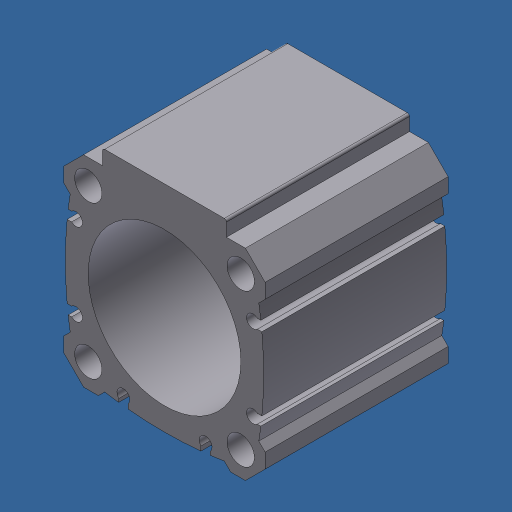
# Autodesk Inventor part: EXTRUSION, CYLINDER, ALUMINIUM, PHD, 50MM
Saved by Autodesk Inventor 2024.3 (Build 283343000, 343)
## iProperties
Manager: _
Category: _
RuleStatus: InUse
Shininess: 64.0
Angle Display Precision: 2
Document Length Units: 11269
Document Angle Units: 11279
Document Time Units: 11290
Document Mass Units: 11283
Document Length Units Precision: 3
Document Angle Units Precision: 2
Part Number: EXTRUSION, CYLINDER, ALUMINIUM, PHD, 50MM
Material: Aluminum, 6061-T6
Document SubType Name: Modeling
Created: 2019-07-31
Designer: -
Manufacturer: Standard
Standards Organization: Custom
Checked By: 00
Engr Approved By: _
User Status: Work In Process
Description: EXTRUSION, CYLINDER, ALUMINIUM, PHD, 50MM
Density: 2.71 g/cm^3
Mass: 328.022 g
Surface Area: 394.618 cm^2
Volume: 121.041 cm^3
Mfg Approved By: -
Appearance: Aluminum (Flat)
BeforeDocSave0: Mass
BeforeDocSave1: PartFinishTrigger
Density: 0.0
Volumn: 0.0
Area: 0.0
PropertySet Name: Model Information
Control State: 0
Master: False
Checked Out: False
CN_MASS: 0.33
CN_SERVICEABLE: _
CL_runCount: 0
FIRST_DESCRIPTION: _
SECOND_DESCRIPTION: _
THIRD_DESCRIPTION: _
Revision Number: A
Subject: _
Author: -
Keywords: -
Autodesk Inventor part; units mm, degrees
ref_plane "YZ Plane" through (0, 0, 0) normal (1, 0, 0) x (0, 1, 0)
ref_plane "XZ Plane" through (0, 0, 0) normal (0, 1, 0) x (-1, 0, 0)
ref_plane "XY Plane" through (0, 0, 0) normal (0, 0, 1) x (1, 0, 0)
sketch "Sketch1" plane through (0, 0, 0) normal (0, 0, 1) x (1, 0, 0)
  line L0 (0, 124.8586) -> (0, -45.1372) projected
  line L1 (-106.1171, 0) -> (141.4895, 0) projected
  line L2 (-32.9946, 26.5288) -> (-32.9946, 21.6916)
  line L3 (-32.9946, 26.5288) -> (-26.5288, 32.9946)
  line L4 (-26.5288, 32.9946) -> (-20.308, 32.9946)
  line L5 (-20.308, 32.9946) -> (-20.308, 37.2864)
  line L6 (-19.596, 37.9984) -> (19.608, 37.9984)
  line L7 (20.32, 37.2864) -> (20.32, 32.9946)
  line L8 (20.32, 32.9946) -> (26.5288, 32.9946)
  line L9 (32.9946, 26.5288) -> (32.9946, 21.6916)
  line L10 (32.9946, 21.6916) -> (30.9118, 19.6088)
  line L11 (-32.9946, 21.6916) -> (-30.9118, 19.6088)
  line L12 (-30.9531, 19.3556) -> (-30.9531, 19.3556)
  line L13 (-31.5752, 15.0241) -> (-30.4686, 15.0241)
  line L14 (-30.9118, -19.6088) -> (-32.9946, -21.6916)
  line L15 (-32.9946, -21.6916) -> (-32.9946, -26.5288)
  line L16 (-32.9946, -26.5288) -> (-26.5288, -32.9946)
  line L17 (-26.5288, -32.9946) -> (-21.6916, -32.9946)
  line L18 (-21.6916, -32.9946) -> (-19.6088, -30.9118)
  line L19 (19.6088, -30.9118) -> (21.6916, -32.9946)
  line L20 (21.6916, -32.9946) -> (26.5288, -32.9946)
  line L21 (26.5288, -32.9946) -> (32.9946, -26.5288)
  line L22 (32.9946, -26.5288) -> (32.9946, -21.6916)
  line L23 (32.9946, -21.6916) -> (30.9118, -19.6088)
  line L24 (31.5752, 15.0241) -> (30.4686, 15.0241)
  line L25 (31.9201, 11.9507) -> (30.4686, 11.9507)
  line L26 (31.9201, -11.9507) -> (30.4686, -11.9507)
  line L27 (31.5752, -15.0241) -> (30.4686, -15.0241)
  line L28 (-30.4686, 11.9507) -> (-31.9201, 11.9507)
  arc A0 (-30.4686, 11.9507) -> (-30.4686, 15.0241) centre (-29.0068, 13.4874) ccw
  arc A1 (-30.4686, -15.0241) -> (-30.4686, -11.9507) centre (-29.0068, -13.4874) ccw
  arc A2 (30.4686, -11.9507) -> (30.4686, -15.0241) centre (29.0068, -13.4874) ccw
  arc A3 (30.4686, 15.0241) -> (30.4686, 11.9507) centre (29.0068, 13.4874) ccw
  line L29 (-30.4686, -15.0241) -> (-31.5752, -15.0241)
  line L30 (-15.0241, -30.4686) -> (-15.0241, -31.5752)
  line L31 (-11.9507, -30.4686) -> (-11.9507, -31.9201)
  line L32 (11.9507, -30.4686) -> (11.9507, -31.9201)
  line L33 (15.0241, -30.4686) -> (15.0241, -31.5752)
  arc A4 (-11.9507, -30.4686) -> (-15.0241, -30.4686) centre (-13.4874, -29.0068) ccw
  arc A5 (15.0241, -30.4686) -> (11.9507, -30.4686) centre (13.4874, -29.0068) ccw
  circle A6 centre (0, 0) radius 25.04
  line L34 (-30.4686, -11.9507) -> (-31.9201, -11.9507)
  arc A7 (30.9118, -19.6088) -> (31.5752, -15.0241) centre (-88.4309, 0) ccw
  arc A8 (31.9201, -11.9507) -> (31.9201, 11.9507) centre (-88.4309, 0) ccw
  arc A9 (31.5752, 15.0241) -> (30.9118, 19.6088) centre (-88.4309, 0) ccw
  line L35 (26.5288, 32.9946) -> (32.9946, 26.5288)
  arc A10 (-19.6088, -30.9118) -> (-15.0241, -31.5752) centre (0, 88.4309) ccw
  arc A11 (-30.9118, 19.6088) -> (-31.5752, 15.0241) centre (88.4309, 0) ccw
  arc A12 (-31.9201, 11.9507) -> (-31.9201, -11.9507) centre (88.4309, 0) ccw
  arc A13 (-31.5752, -15.0241) -> (-30.9118, -19.6088) centre (88.4309, 0) ccw
  arc A14 (-11.9507, -31.9201) -> (11.9507, -31.9201) centre (0, 88.4309) ccw
  arc A15 (15.0241, -31.5752) -> (19.6088, -30.9118) centre (0, 88.4309) ccw
  arc A16 (-19.596, 37.9984) -> (-20.308, 37.2864) centre (-19.596, 37.2864) ccw
  arc A17 (20.32, 37.2864) -> (19.608, 37.9984) centre (19.608, 37.2864) ccw
  dimension "d0" = 4.2418
  dimension "d1" = 50.08
  dimension "d3" = 0.712
  constraints: 68 end point, 34 point on circle, 18 centre point, 13 horizontal, 10 coincident, 10 vertical, 6 equal radius, 4 tangent, 1 parallel, 1 point on line, 28 other
  measures "d0" diameter of A0
  measures "d1" diameter of A6
  measures "d3" radius of A16
extrude "PHD, 50MM" add sketch "Sketch1" against normal blind 60 contours L6 A17 L7 L8 L35 L9 L10 A9 L24 A3 L25 A8 L1 A6 L0 | L0 A6 L1 A12 L28 A0 L13 A11 L11 L2 L3 L4 L5 A16 L6 | L1 A8 L26 A2 L27 A7 L23 L22 L21 L20 L19 A15 L33 A5 L32 A14 L0 A6 | A6 L0 A14 L31 A4 L30 A10 L18 L17 L16 L15 L14 A13 L29 A1 L34 A12 L1
sketch "Sketch2" plane through (0, 0, 0) normal (0, 0, 1) x (1, 0, 0)
  line L0 (0, 59.2963) -> (0, -40.0939) projected
  line L1 (-39.5935, 0) -> (52.7914, 0) projected
  point P0 (-25, 25)
  point P1 (25, 25)
  point P2 (25, -25)
  point P3 (-25, -25)
  dimension "d6" = 25
  dimension "d7" = 25
  dimension "d8" = 25
  dimension "d9" = 25
  constraints: 2 horizontal alignment, 2 vertical alignment
  measures "d6" distance from line of point (-25, 25) L0
  measures "d7" distance from line of point (25, 25) L0
  measures "d8" distance from line of point (-25, 25) L1
  measures "d9" distance from line of point (-25, -25) L1
hole "Hole1" at (-25, 25, 0) at (25, 25, 0) at (25, -25, 0) at (-25, -25, 0) direction (0, 0, -1) diameter 9 end through all
equation "\"d7\" = d6"
equation "\"d8\" = d6"
equation "\"d9\" = d6"
